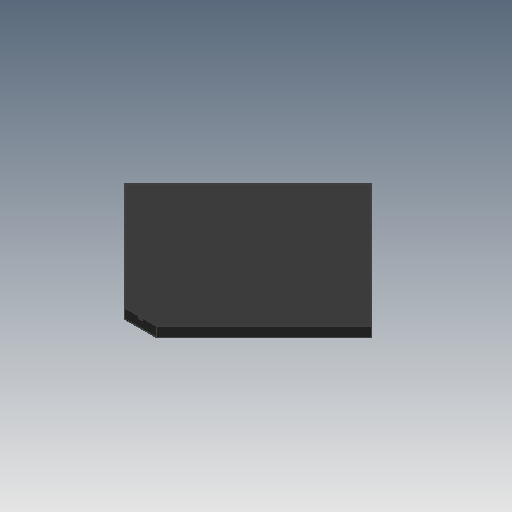
# Autodesk Inventor part: rubberizedCoating
Saved by Autodesk Inventor 2020 (Build 240168000, 168)
## iProperties
Created: 2016-02-15
Part Number: rubberizedCoating
Material: Rubber
Document SubType Name: Modeling
Designer: sawai
Density: 0.93 g/cm^3
Appearance: Rubber - Black
Author: sawai
Autodesk Inventor part; units mm, degrees
note: some values were not read from the file. Left out: dimensions or parameters whose unit could not be read.
ref_plane "YZ Plane" through (0, 0, 0) normal (1, 0, 0) x (0, 1, 0)
ref_plane "XZ Plane" through (0, 0, 0) normal (0, 1, 0) x (-1, 0, 0)
ref_plane "XY Plane" through (0, 0, 0) normal (0, 0, 1) x (1, 0, 0)
sketch "Sketch1" plane through (0, 0, 0) normal (0, 0, 1) x (1, 0, 0)
  line L0 (-141.7042, 0) -> (-17.9605, 123.7437)
  line L1 (17.9605, 123.7437) -> (141.7042, 0)
  line L2 (141.7042, 0) -> (0, -141.7042)
  line L3 (0, -141.7042) -> (-141.7042, 0)
  line L4 (-141.7042, 0) -> (141.7042, 0) construction
  line L5 (0, 141.7042) -> (0, -141.7042) construction
  line L6 (17.9605, 123.7437) -> (-17.9605, 123.7437)
  line L7 (-18.1709, 124.2517) -> (18.1709, 124.2517)
  line L8 (18.1709, 124.2517) -> (142.4226, 0)
  line L9 (142.4226, 0) -> (0, -142.4226)
  line L10 (0, -142.4226) -> (-142.4226, 0)
  line L11 (-142.4226, 0) -> (-18.1709, 124.2517)
  point P0 (0, 0)
  dimension "d0" = 200.4
  dimension "d1" = 200.4
  dimension "d7" = 25.4
  dimension "d8" = 25.4
  dimension "d9" = 0.508
  constraints: 24 end point, 4 parallel, 2 midpoint, 2 perpendicular, 2 point on line, 1 horizontal, 4 other
  measures "d0" distance of L5.start L1.end
  measures "d1" distance between parallel lines of L3 L1
  measures "d7" distance of L1.start L5.start
  measures "d8" distance of L0.end L5.start
  measures "d9" distance between parallel lines of L0 L11
extrude "Extrusion1" add sketch "Sketch1" along normal mid plane 10.4
sketch "Sketch4" plane through (-18.1709, 124.2517, 5.2) normal (0, 1, 0) x (1, 0, 0)
  line L0 (20.1709, 0) -> (16.1709, 0)
  line L1 (16.1709, 0) -> (16.1709, 2)
  line L2 (16.1709, 2) -> (20.1709, 2)
  line L3 (20.1709, 2) -> (20.1709, 0)
  line L4 (36.3419, 0) -> (0, 0) projected
  point P0 (18.1709, 5.2)
  point P1 (18.1709, 0)
  dimension "d16" = 4
  dimension "d17" = 2
  constraints: 8 end point, 2 midpoint, 2 parallel, 1 horizontal, 1 perpendicular
  measures "d16" distance of L1.end L2.end
  measures "d17" distance of L0.end L1.end
extrude "Extrusion3" cut sketch "Sketch4" against normal up to surface (0.508 mm away)
sketch "Sketch2" plane through (0, 0, 5.2) normal (0, 0, 1) x (1, 0, 0)
  line L0 (142.4226, 0) -> (0, -142.4226) projected
  line L1 (18.1709, 124.2517) -> (142.4226, 0) projected
  line L2 (-18.1709, 124.2517) -> (18.1709, 124.2517) projected
  line L3 (-142.4226, 0) -> (-18.1709, 124.2517) projected
  line L4 (0, -142.4226) -> (-142.4226, 0) projected
extrude "Extrusion2" add sketch "Sketch2" along normal blind 0.508
mirror "Mirror1" about plane through (0, 0, 0) normal (0, 0, 1) of "Extrusion2"
equation "\"d0\" = ScintillatorWidth + 2 * silveringThickness"
equation "\"d1\" = ScintillatorHeight + 2 * silveringThickness"
equation "\"d7\" = cornerChamfer"
equation "\"d8\" = d7"
equation "\"d9\" = rubberizedCoating"
equation "\"d3\" = ScintillatorThickness + 2 * silveringThickness"
equation "\"d5\" = rubberizedCoating"
equation "\"OpticalFiberClearence\" = 0.15"
equation "\"ScintillatorEdgeClearence\" = 3"
equation "\"ShallowTrackDepth\" = 1.3"
equation "\"DeepTrackDepth\" = 5.571"
equation "\"FiberEdgeOffsett\" = 5"
equation "\"LoopLargeTrackRatio\" = 1.5"
equation "\"FiberSensorClerence\" = 0.5"
equation "\"MountingScrewOffsett\" = 9"
equation "\"FoilThickness\" = 0.2"
equation "\"silveringThickness\" = 0.2"
equation "\"mppcMountDepth\" = 6.35"
equation "\"opticalFiberClearence\" = 0.071"
equation "\"scintillatorEdgeClearence\" = 3"
equation "\"fiberEdgeOffsett\" = 5"
equation "\"shallowTrackDepth\" = 1.142"
equation "\"deepTrackDepth\" = 5.571"
equation "\"opticalFiberDiameter\" = 1"
equation "\"mountingSpacing\" = 18"
equation "\"cornerChamfer\" = 25.4"
equation "\"SmallTrackDiameter\" = 175"
equation "\"ScintillatorWidth\" = 200"
equation "\"ScintillatorHeight\" = 200"
equation "\"ScintillatorThickness\" = 10"
body "Solid1"
